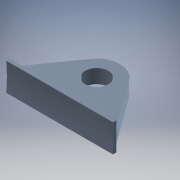
# Autodesk Inventor part: Lifting Lug
Saved by Autodesk Inventor 2016 (Build 200138000, 138)
## iProperties
Created: 2018-11-07
Part Number: Lifting Lug
Material: Steel ASTM A36
Document SubType Name: Modeling
Designer: asus
Density: 7.85 g/cm^3
Appearance: Steel Blue
Mass: 536.653 g
Surface Area: 176.425 cm^2
Volume: 68.3634 cm^3
Author: asus
Autodesk Inventor part; units mm, degrees
ref_plane "YZ Plane" through (0, 0, 0) normal (1, 0, 0) x (0, 1, 0)
ref_plane "XZ Plane" through (0, 0, 0) normal (0, 1, 0) x (-1, 0, 0)
ref_plane "XY Plane" through (0, 0, 0) normal (0, 0, 1) x (1, 0, 0)
sketch "Sketch1" plane through (0, 0, 0) normal (0, 0, 1) x (1, 0, 0)
  line L0 (0, 0) -> (-57, 0)
  line L1 (0, 0) -> (58, 0)
  circle A0 centre (0, 40) radius 12.5
  arc A1 (20.1852, 54.7498) -> (-20.3716, 54.4913) centre (0, 40) ccw
  line L2 (-57, 0) -> (-57, 3)
  line L3 (-57, 3) -> (-20.3716, 54.4913)
  line L4 (58, 0) -> (58, 3)
  line L5 (58, 3) -> (20.1852, 54.7498)
  line L6 (-57, 3) -> (58, 3)
  point P0 (29, 0)
  dimension "d0" = 57
  dimension "d1" = 58
  dimension "d3" = 25
  dimension "d4" = 50
  dimension "d5" = 40
  dimension "d6" = 3
  dimension "d7" = 3
  constraints: 14 end point, 3 coincident, 2 centre point, 2 point on circle, 2 tangent, 1 horizontal, 1 horizontal alignment, 1 midpoint, 1 parallel, 1 vertical, 1 vertical alignment
  measures "d0" distance of L0.start L0.end
  measures "d1" distance of L0.start L1.end
  measures "d3" diameter of A0
  measures "d4" diameter of A1
  measures "d5" distance of point (0, 0) A0.centre
  measures "d6" distance of L1.end L4.end
  measures "d7" distance of L0.end L2.end
extrude "Extrusion1" add sketch "Sketch1" along normal mid plane 15 contours L3 A1 L5 L6
sketch "Sketch2" plane through (0, 0, 0) normal (0, 0, 1) x (1, 0, 0)
  line L0 (-57, 3) -> (58, 3) projected
  line L1 (-57, 3) -> (-57, 0)
  line L2 (-57, 0) -> (58, 0)
  line L3 (58, 0) -> (58, 3)
  point P0 (0, 0)
  point P1 (0.5, 0)
  constraints: 6 end point, 2 perpendicular, 1 horizontal alignment, 1 midpoint, 1 vertical
extrude "Extrusion2" add sketch "Sketch2" along normal mid plane 30
sketch "Sketch3" plane through (58, 0, 15) normal (1, 0, 0) x (0, 0, -1)
  arc A0 (30, -0.6339) -> (0, -0.6339) centre (15, -177.8) ccw
  line L0 (0, 0) -> (30, 0) projected
  line L1 (30, 0) -> (30, -0.6339)
  line L2 (0, 0) -> (0, -0.6339)
  point P0 (15, 0)
  point P1 (15, 0)
  dimension "d13" = 355.6
  constraints: 4 end point, 3 point on circle, 2 parallel, 1 centre point, 1 midpoint, 1 vertical
  measures "d13" diameter of A0
extrude "Extrusion3" add sketch "Sketch3" against normal up to surface (115 mm away)
body "Solid1"
